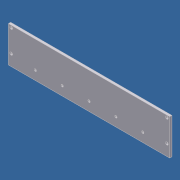
# Autodesk Inventor part: Bottom
Saved by Autodesk Inventor 2012 SP1 (Build 160190100, 190)
## iProperties
Created: 2010-12-14
Part Number: Bottom
Document SubType Name: Modeling
Designer: berny
Density: 2.71 g/cm^3
Material: Aluminum-6061
Mass: 790.52 g
Surface Area: 1009.94 cm^2
Volume: 291.705 cm^3
Author: berny
Autodesk Inventor part; units mm, degrees
ref_plane "YZ Plane" through (0, 0, 0) normal (1, 0, 0) x (0, 1, 0)
ref_plane "XZ Plane" through (0, 0, 0) normal (0, 1, 0) x (-1, 0, 0)
ref_plane "XY Plane" through (0, 0, 0) normal (0, 0, 1) x (1, 0, 0)
sketch "Sketch1" plane through (0, 0, 0) normal (0, 0, 1) x (1, 0, 0)
  line L0 (0, 0) -> (457.2, 0)
  line L1 (457.2, 0) -> (457.2, 101.6)
  line L2 (457.2, 101.6) -> (0, 101.6)
  line L3 (0, 101.6) -> (0, 0)
  dimension "d0" = 101.6
  dimension "d1" = 457.2
  constraints: 8 end point, 2 parallel, 1 horizontal, 1 perpendicular
  measures "d0" distance of L2.end L0.start
  measures "d1" distance of L0.start L0.end
extrude "Extrusion1" add sketch "Sketch1" along normal blind 6.35
sketch "Sketch2" plane through (0, 0, 6.35) normal (0, 0, 1) x (1, 0, 0)
  line L0 (0, 0) -> (0, 101.6) projected
  line L1 (457.2, 0) -> (0, 0) projected
  line L2 (457.2, 101.6) -> (457.2, 0) projected
  point P0 (449.2625, 31.75)
  point P1 (449.2625, 95.25)
  point P2 (7.9375, 31.75)
  point P3 (7.9375, 95.25)
  dimension "d4" = 31.75
  dimension "d5" = 6.35
  dimension "d6" = 7.9375
  dimension "d7" = 7.9375
  constraints: 2 horizontal alignment, 2 vertical alignment
  measures "d4" distance from line of L1 point (449.262, 31.75)
  measures "d5" vertical distance of L2.start point (449.262, 95.25)
  measures "d6" distance from line of L2 point (449.262, 31.75)
  measures "d7" distance from line of L0 point (7.937, 31.75)
hole "Hole1" at (449.2625, 31.75, 6.35) at (449.2625, 95.25, 6.35) at (7.9375, 31.75, 6.35) at (7.9375, 95.25, 6.35) direction (0, 0, -1) diameter 4.318 end through all counterbore diameter 7.9502 counterbore depth 4.1656 clearance for "Socket Head Cap Screw" size "#8" standard "Ansi Unified Screw Threads"
sketch "Sketch3" plane through (0, 0, 0) normal (0, 0, -1) x (-1, 0, 0)
  line L0 (0, 0) -> (-457.2, 0) projected
  line L1 (0, 101.6) -> (0, 0) projected
  point P0 (-76.2, 25.4)
  point P1 (-228.6, 25.4)
  point P2 (-381, 25.4)
  point P3 (-152.4, 25.4)
  point P4 (-304.8, 25.4)
  dimension "d15" = 76.2
  dimension "d16" = 25.4
  dimension "d17" = 152.4
  dimension "d18" = 152.4
  dimension "d26" = 76.2
  dimension "d27" = 25.4
  dimension "d28" = 76.2
  constraints: 3 horizontal alignment
  measures "d15" distance from line of point (-76.2, 25.4) L1
  measures "d16" distance from line of L0 point (-76.2, 25.4)
  measures "d17" distance of point (-228.6, 25.4) point (-76.2, 25.4)
  measures "d18" distance of point (-381, 25.4) point (-228.6, 25.4)
  measures "d26" distance of point (-152.4, 25.4) point (-76.2, 25.4)
  measures "d27" distance from line of L0 point (-304.8, 25.4)
  measures "d28" distance of point (-228.6, 25.4) point (-304.8, 25.4)
hole "Hole2" at (76.2, 25.4, 0) at (228.6, 25.4, 0) at (381, 25.4, 0) direction (0, 0, 1) diameter 6.7564 end through all counterbore diameter 11.1252 counterbore depth 3.81 clearance for "Socket Head Cap Screw" size "1/4" standard "Ansi Unified Screw Threads"
sketch "Sketch4" plane through (0, 0, 0) normal (0, 0, -1) x (-1, 0, 0)
  circle A0 centre (-228.6, 25.4) radius 5.5626 projected
  circle A1 centre (-76.2, 25.4) radius 5.5626 projected
  point P0 (-152.4, 25.4)
  point P1 (-304.8, 25.4)
  dimension "d29" = 76.2
  dimension "d30" = 76.2
  constraints: 2 horizontal alignment
  measures "d29" distance of point (-152.4, 25.4) A1.centre
  measures "d30" distance of point (-304.8, 25.4) A0.centre
hole "Hole3" at (152.4, 25.4, 0) at (304.8, 25.4, 0) direction (0, 0, 1) diameter 6.7564 depth 25.4 tip angle 118 counterbore diameter 11.1252 counterbore depth 3.81 clearance for "Socket Head Cap Screw" size "1/4" standard "Ansi Unified Screw Threads"
body "Solid1"
